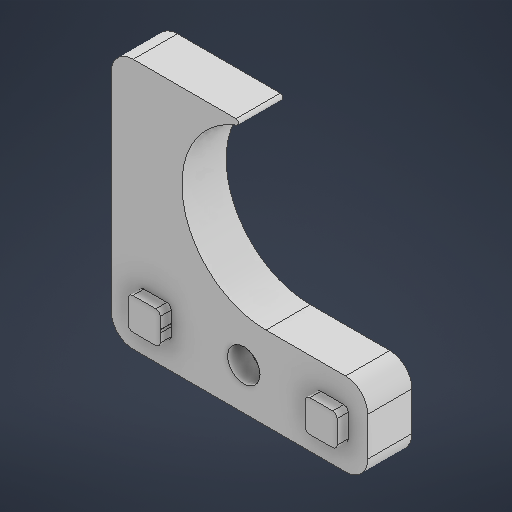
# Autodesk Inventor part: piston holder for goal rush
Saved by Autodesk Inventor 2025.1 (Build 291241000, 241)
## iProperties
Created: 2025-01-21
Part Number: piston holder for goal rush
Material: Generic
Document SubType Name: Modeling
Designer: Juanl
Density: 1 g/cm^3
Appearance: Default
Author: Juanl
Autodesk Inventor part; units mm, degrees
ref_plane "YZ Plane" through (0, 0, 0) normal (1, 0, 0) x (0, 1, 0)
ref_plane "XZ Plane" through (0, 0, 0) normal (0, 1, 0) x (-1, 0, 0)
ref_plane "XY Plane" through (0, 0, 0) normal (0, 0, 1) x (1, 0, 0)
sketch "Sketch1" plane through (0, 0, 0) normal (0, 0, 1) x (1, 0, 0)
  line L0 (-18.415, 5.9563) -> (18.415, 5.9563)
  line L1 (18.415, 5.9563) -> (18.415, -5.9563)
  line L2 (18.415, -5.9563) -> (-18.415, -5.9563)
  line L3 (-18.415, -5.9563) -> (-18.415, 5.9563)
  line L4 (-18.415, 5.9563) -> (18.415, -5.9563) construction
  line L5 (18.415, 5.9563) -> (-18.415, -5.9563) construction
  point P0 (0, 0)
  dimension "d0" = 36.83
  dimension "d1" = 11.9126
  constraints: 12 end point, 2 midpoint, 2 parallel, 1 horizontal, 1 perpendicular
  measures "d0" distance of L1.end L2.end
  measures "d1" distance of L2.end L0.start
extrude "Extrusion1" add sketch "Sketch1" along normal blind 6.35
sketch "Sketch2" plane through (0, 0, 6.35) normal (0, 0, 1) x (1, 0, 0)
  line L0 (-18.415, 5.9563) -> (-18.415, -5.9563) projected
  line L1 (-18.415, 0) -> (18.415, 0)
  line L2 (18.415, -5.9563) -> (18.415, 5.9563) projected
  line L3 (-18.415, 0) -> (-20.6375, 0)
  line L4 (-18.415, 0) -> (-12.065, 0)
  circle A0 centre (-12.065, 0) radius 2.3241
  circle A1 centre (0.635, 0) radius 2.3241
  circle A2 centre (13.335, 0) radius 2.3241
  line L5 (-13.716, 2.286) -> (-10.414, 2.286)
  line L6 (-9.779, 1.651) -> (-9.779, -1.651)
  line L7 (-10.414, -2.286) -> (-13.716, -2.286)
  line L8 (-14.351, -1.651) -> (-14.351, 1.651)
  line L9 (-14.351, 2.286) -> (-9.779, -2.286) construction
  line L10 (-9.779, 2.286) -> (-14.351, -2.286) construction
  line L11 (11.684, 2.286) -> (14.986, 2.286)
  line L12 (15.621, 1.651) -> (15.621, -1.651)
  line L13 (14.986, -2.286) -> (11.684, -2.286)
  line L14 (11.049, -1.651) -> (11.049, 1.651)
  line L15 (11.049, 2.286) -> (15.621, -2.286) construction
  line L16 (15.621, 2.286) -> (11.049, -2.286) construction
  arc A3 (-13.716, 2.286) -> (-14.351, 1.651) centre (-13.716, 1.651) ccw
  arc A4 (-9.779, 1.651) -> (-10.414, 2.286) centre (-10.414, 1.651) ccw
  arc A5 (-10.414, -2.286) -> (-9.779, -1.651) centre (-10.414, -1.651) ccw
  arc A6 (-14.351, -1.651) -> (-13.716, -2.286) centre (-13.716, -1.651) ccw
  arc A7 (11.684, 2.286) -> (11.049, 1.651) centre (11.684, 1.651) ccw
  arc A8 (15.621, 1.651) -> (14.986, 2.286) centre (14.986, 1.651) ccw
  arc A9 (14.986, -2.286) -> (15.621, -1.651) centre (14.986, -1.651) ccw
  arc A10 (11.049, -1.651) -> (11.684, -2.286) centre (11.684, -1.651) ccw
  point P0 (0, 0)
  point P1 (-9.779, -0.4191)
  point P2 (-9.7409, 0)
  point P3 (-9.779, 0)
  dimension "d5" = 6.35
  dimension "d6" = 4.6482
  dimension "d9" = 12.7
  dimension "d16" = 4.572
  dimension "d17" = 4.572
  dimension "d18" = 4.572
  dimension "d19" = 4.572
  dimension "d20" = 0.635
  constraints: 30 end point, 18 point on line, 16 point on circle, 16 tangent, 11 centre point, 7 equal radius, 6 midpoint, 4 parallel, 3 horizontal, 2 perpendicular, 1 coincident, 4 other
  measures "d5" distance of L1.start L4.end
  measures "d6" diameter of A0
  measures "d9" distance of A0.centre A1.centre
  measures "d16" distance between parallel lines of L7 L5
  measures "d17" distance between parallel lines of L6 L8
  measures "d18" distance of L15.end L16.end
  measures "d19" distance between parallel lines of L13 L11
  measures "d20" radius of A3
extrude "Extrusion2" add sketch "Sketch2" along normal blind 1.5875 contours L8 A0 L5 L6 L1 | L1 L6 A0 L7 L8 | L8 A3 L5 A0 | A0 L7 A6 L8 | L1 A0 L6 | L5 A4 L6 A0 | A0 L6 A5 L7 | L14 A2 L11 L12 L1 | L1 L12 A2 L13 L14 | L14 A7 L11 A2 | A2 L13 A10 L14 | A2 L11 A8 L12 | L12 A9 L13 A2 picked at (-9.772, -0.2331)
extrude "Extrusion3" cut sketch "Sketch2" against normal through all contours A1 L1 | L1 A1
sketch "Sketch9" plane through (-18.415, 5.9563, 0) normal (0, 1, 0) x (1, 0, 0)
  line L0 (0, 0) -> (36.83, 0) projected
  line L1 (0, -6.35) -> (36.83, -6.35) projected
  line L2 (0, 0) -> (22.225, 0)
  line L3 (22.225, 0) -> (22.225, -6.35)
  line L4 (22.225, -6.35) -> (0, -6.35)
  line L5 (0, -6.35) -> (0, 0)
  point P0 (18.415, 0)
  dimension "d45" = 22.225
  constraints: 8 end point, 2 parallel, 1 horizontal, 1 perpendicular, 1 point on line
  measures "d45" distance of L3.end L4.end
extrude "Extrusion9" add sketch "Sketch9" along normal blind 24.13
sketch "Sketch10" plane through (0, 0, 0) normal (0, 0, -1) x (-1, 0, 0)
  line L0 (-18.415, 5.9563) -> (-3.81, 5.9563) projected
  line L1 (18.415, 30.0863) -> (-3.81, 30.0863) projected
  arc A0 (-3.81, 5.9563) -> (-3.81, 30.0863) centre (-3.81, 18.0213) ccw
  line L2 (-3.81, 30.0863) -> (-3.81, 5.9563)
  point P0 (0, 0)
  constraints: 2 end point, 2 point on circle, 1 centre point, 1 vertical
extrude "Extrusion10" cut sketch "Sketch10" against normal blind 19.05
fillet "Fillet7" radius 0.381 1 edges at (3.81, 30.0863, 3.175)
fillet "Fillet8" radius 3.175 4 edges at (-18.415, 30.0863, 3.175) (18.415, 5.9563, 3.175) (18.415, -5.9563, 3.175) (-18.415, -5.9563, 3.175)
sketch "Sketch11" plane through (0, 0, 0) normal (0, 0, -1) x (-1, 0, 0)
  circle A0 centre (-0.635, 0) radius 2.3241 projected
  circle A1 centre (-0.635, 0) radius 4.1275
  point P0 (0, 0)
  dimension "d52" = 8.255
  constraints: 1 centre point, 1 coincident
  measures "d52" diameter of A1
extrude "Extrusion11" cut sketch "Sketch11" against normal blind 3.175
body "Solid1"
